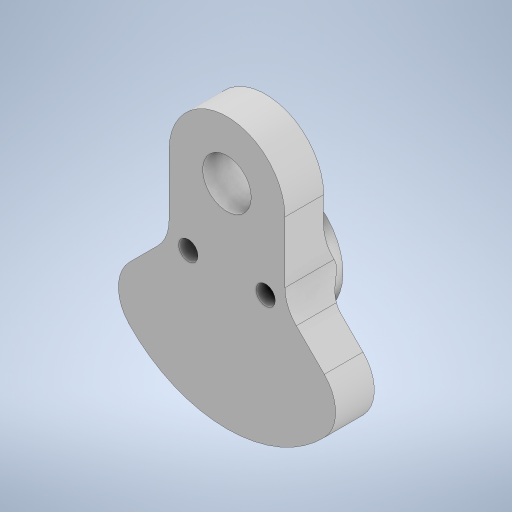
# Autodesk Inventor part: Crank on Crankshaft
Saved by Autodesk Inventor 2023 (Build 270158000, 158)
## iProperties
Created: 2022-10-29
Part Number: Crank on Crankshaft
Material: Generic
Document SubType Name: Modeling
Designer: tommy
Density: 1 g/cm^3
Appearance: Default
Author: tommy
## iProperties of the stored document Crank on Crankshaft_3DPrint.ipt
Created: 2022-10-29
Part Number: Crank on Crankshaft_3DPrint
Material: Generic
Document SubType Name: Modeling
Designer: tommy
Density: 1 g/cm^3
Appearance: Default
Author: tommy
Autodesk Inventor part; units mm, degrees
ref_plane "YZ Plane" through (0, 0, 0) normal (1, 0, 0) x (0, 1, 0)
ref_plane "XZ Plane" through (0, 0, 0) normal (0, 1, 0) x (-1, 0, 0)
ref_plane "XY Plane" through (0, 0, 0) normal (0, 0, 1) x (1, 0, 0)
sketch "Sketch1" plane through (0, 0, 0) normal (0, 0, 1) x (1, 0, 0)
  circle A0 centre (0, 12.7) radius 3.9878
  line L0 (-11.384872, -1.859872) -> (-13.738625, -4.213625)
  line L1 (11.384872, -1.859872) -> (13.738625, -4.213625)
  circle A1 centre (-6.35, 0) radius 1.5875
  circle A2 centre (6.35, 0) radius 1.5875
  line L2 (-9.525, 2.630256) -> (-9.525, 12.7)
  line L3 (9.525, 2.630256) -> (9.525, 12.7)
  arc A3 (9.525, 12.7) -> (-9.525, 12.7) centre (0, 12.7) ccw
  arc A4 (9.525, 12.7) -> (-9.525, 12.7) centre (0, 12.7) ccw
  arc A5 (-16.092142, -15.329501) -> (16.092142, -15.329501) centre (0, 0) ccw
  line L4 (-11.384872, -1.859872) -> (-15.984515, -6.459515)
  line L5 (11.384872, -1.859872) -> (15.984515, -6.459515)
  arc A6 (-15.984515, -6.459515) -> (-16.092142, -15.329501) centre (-11.494387, -10.949643) ccw
  arc A7 (16.092142, -15.329501) -> (15.984515, -6.459515) centre (11.494387, -10.949643) ccw
  arc A8 (-11.384872, -1.859872) -> (-9.525, 2.630256) centre (-15.875, 2.630256) ccw
  arc A9 (9.525, 2.630256) -> (11.384872, -1.859872) centre (15.875, 2.630256) ccw
  arc A10 (-4.611271, 8.334375) -> (4.611271, 8.334375) centre (0, 12.7) ccw
  arc A11 (-4.611271, 8.334375) -> (4.611271, 8.334375) centre (0, 0) ccw
  point P0 (0, 19.05)
  point P1 (-9.525, 0)
  point P2 (-17.362891, -7.837891)
  point P3 (9.525, 0)
  point P4 (17.362891, -7.837891)
  point P5 (-19.738945, -10.213945)
  point P6 (19.738945, -10.213945)
  dimension "d20" = 7.9756
  dimension "d34" = 44.45
  dimension "d35" = 6.35
  dimension "d36" = 6.35
  dimension "d38" = 12.7
  constraints: 20 point on circle, 12 centre point, 12 end point, 9 tangent, 8 point on line, 4 coincident, 2 equal radius, 1 parallel, 1 vertical
  measures "d20" diameter of A0
  measures "d34" diameter of A5
  measures "d35" radius of A6
  measures "d36" radius of A8
  measures "d38" diameter of A10
extrude "Extrusion2" add sketch "Sketch1" along normal blind 6.35 contours A8 L2 A3 L3 A9 L1 L5 A7 A5 A6 L4 L0 | A10 A11
extrude "Extrusion3" add sketch "Sketch1" against normal blind 3.175 contours A10 A11
fillet "Fillet1" radius 3.175 1 edges at (0, -9.525, 0)
body "Solid2"
